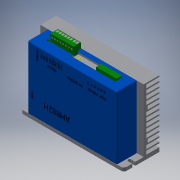
# Autodesk Inventor part: AM882
Saved by Autodesk Inventor 2016 (Build 200138000, 138)
## iProperties
Created: 2015-09-27
Part Number: AM882
Material: Generic
Document SubType Name: Modeling
Density: 1 g/cm^3
Appearance: Default
Autodesk Inventor part; units mm, degrees
ref_plane "YZ Plane" through (0, 0, 0) normal (1, 0, 0) x (0, 1, 0)
ref_plane "XZ Plane" through (0, 0, 0) normal (0, 1, 0) x (-1, 0, 0)
ref_plane "XY Plane" through (0, 0, 0) normal (0, 0, 1) x (1, 0, 0)
sketch "Sketch1" plane through (0, 0, 0) normal (0, 0, 1) x (1, 0, 0)
  line L0 (75.5, -37.5) -> (-75.5, -37.5)
  line L1 (-71.5, 14.5) -> (71.5, 14.5)
  arc A0 (-69.5, -2.25) -> (-69.5, 2.25) centre (-69.5, 0) ccw
  arc A1 (69.5, 2.25) -> (69.5, -2.25) centre (69.5, 0) ccw
  line L2 (-69.5, 2.25) -> (-75.5, 2.25)
  line L3 (-69.5, -2.25) -> (-75.5, -2.25)
  line L4 (69.5, 2.25) -> (75.5, 2.25)
  line L5 (69.5, -2.25) -> (75.5, -2.25)
  line L6 (75.5, 10.5) -> (75.5, 2.25)
  line L7 (75.5, -2.25) -> (75.5, -33.5)
  line L8 (-75.5, -37.5) -> (-75.5, -2.25)
  line L9 (-75.5, 2.25) -> (-75.5, 10.5)
  arc A2 (-71.5, 14.5) -> (-75.5, 10.5) centre (-71.5, 10.5) ccw
  arc A3 (75.5, 10.5) -> (71.5, 14.5) centre (71.5, 10.5) ccw
  line L10 (75.5, -2.25) -> (75.5, -37.5)
  point P0 (0, 0)
  dimension "d1" = 14.5
  dimension "d4" = 52
  dimension "d6" = 4.5
  dimension "d7" = 4.5
  dimension "d8" = 69.5
  dimension "d9" = 69.5
  dimension "d10" = 4
  dimension "d94" = 6
  dimension "d95" = 6
  constraints: 22 end point, 10 perpendicular, 8 point on circle, 8 tangent, 5 parallel, 4 centre point, 1 horizontal, 1 point on line
  measures "d1" distance from line of L1 point (0, 0)
  measures "d4" distance between parallel lines of L0 L1
  measures "d6" diameter of A0
  measures "d7" diameter of A1
  measures "d8" distance of point (0, 0) A1.centre
  measures "d9" distance of point (0, 0) A0.centre
  measures "d10" radius of A2
  measures "d94" distance from line of L9 A0.centre
  measures "d95" distance from line of L6 A1.centre
extrude "Extrusion1" add sketch "Sketch1" along normal blind 5
sketch "Sketch2" plane through (0, 0, 5) normal (0, 0, 1) x (1, 0, 0)
  line L0 (-75.5, -37.5) -> (-75.5, -2.25) projected
  arc A0 (69.5, 2.25) -> (69.5, -2.25) centre (69.5, 0) ccw projected
  line L1 (75.5, 10.5) -> (75.5, 2.25) projected
  line L2 (-71.5, 14.5) -> (71.5, 14.5) projected
  line L3 (-75.5, 2.25) -> (-75.5, 10.5) projected
  line L4 (-65.5, -14.5) -> (-65.5, 14.5)
  line L5 (65.5, -14.5) -> (65.5, 14.5)
  line L6 (-75.5, -14.5) -> (-65.5, -14.5)
  line L7 (65.5, -14.5) -> (75.5, -14.5)
  line L8 (75.5, -14.5) -> (75.5, -37.5)
  line L9 (-75.5, -14.5) -> (-75.5, -37.5)
  line L10 (-75.5, -37.5) -> (75.5, -37.5)
  point P0 (-71.5, -37.5)
  point P1 (0, 0)
  dimension "d13" = 14.5
  dimension "d15" = 10
  dimension "d16" = 10
  constraints: 14 end point, 3 perpendicular, 3 point on line, 1 parallel, 1 vertical
  measures "d13" distance from line of L2 A0.centre
  measures "d15" distance between parallel lines of L5 L1
  measures "d16" distance between parallel lines of L3 L4
extrude "Extrusion2" add sketch "Sketch2" along normal blind 92
sketch "Sketch3" plane through (0, 0, 97) normal (0, 0, 1) x (1, 0, 0)
  line L0 (65.5, 14.5) -> (65.5, -14.5) projected
  line L1 (-65.5, 14.5) -> (65.5, 14.5) projected
  line L2 (-65.5, -14.5) -> (-65.5, 14.5) projected
  line L3 (-65.5, -14.5) -> (65.5, -14.5)
  point P0 (0, 0)
  constraints: 2 end point, 1 perpendicular
extrude "Extrusion3" cut sketch "Sketch3" against normal blind 0.1
sketch "Sketch4" plane through (-71.5, 14.5, 0) normal (0, 1, 0) x (1, 0, 0)
  line L0 (6, -96.9) -> (137, -96.9) projected
  line L1 (137, -5) -> (137, -96.9) projected
  line L2 (0, -5) -> (143, -5) projected
  line L3 (6, -5) -> (6, -96.9) projected
  line L4 (6, -5) -> (137, -5)
  point P0 (71.5, 0)
  constraints: 2 end point, 1 collinear
extrude "Extrusion4" cut sketch "Sketch4" against normal blind 0.1
fillet "Fillet3" radius 2 5 edges at (-65.5, -0.05, 96.9) (0, 14.4, 96.9) (-65.5, 14.4, 50.95) (65.5, 14.4, 50.95) (65.5, -0.05, 96.9)
sketch "Sketch5" plane through (75.5, -37.5, 0) normal (1, 0, 0) x (0, 0, -1)
  line L0 (-5, 23.1496) -> (-97, 23.1496)
  line L1 (-0.1332, -0.4244) -> (-97.1332, -0.4244)
  line L2 (-95, -0.4244) -> (-90, -0.4244)
  line L3 (-90, -0.4244) -> (-90, 19.1496)
  line L4 (-90, 19.1496) -> (-95, 19.1496)
  line L5 (-95, 19.1496) -> (-95, -0.4244)
  line L6 (-97, 23.1496) -> (-97, 4.1496)
  line L7 (-88, -0.4244) -> (-83, -0.4244)
  line L8 (-83, -0.4244) -> (-83, 19.1496)
  line L9 (-83, 19.1496) -> (-88, 19.1496)
  line L10 (-88, 19.1496) -> (-88, -0.4244)
  line L11 (-76, -0.4244) -> (-81, -0.4244)
  line L12 (-81, -0.4244) -> (-81, 19.1496)
  line L13 (-81, 19.1496) -> (-76, 19.1496)
  line L14 (-76, 19.1496) -> (-76, -0.4244)
  line L15 (-69, -0.4244) -> (-74, -0.4244)
  line L16 (-74, -0.4244) -> (-74, 19.1496)
  line L17 (-74, 19.1496) -> (-69, 19.1496)
  line L18 (-69, 19.1496) -> (-69, -0.4244)
  line L19 (-67, -0.4244) -> (-62, -0.4244)
  line L20 (-62, -0.4244) -> (-62, 17.1496)
  line L21 (-62, 17.1496) -> (-67, 17.1496)
  line L22 (-67, 17.1496) -> (-67, -0.4244)
  line L23 (-55, -0.4244) -> (-60, -0.4244)
  line L24 (-60, -0.4244) -> (-60, 19.1496)
  line L25 (-60, 19.1496) -> (-55, 19.1496)
  line L26 (-55, 19.1496) -> (-55, -0.4244)
  line L27 (-48, -0.4244) -> (-53, -0.4244)
  line L28 (-53, -0.4244) -> (-53, 19.1496)
  line L29 (-53, 19.1496) -> (-48, 19.1496)
  line L30 (-48, 19.1496) -> (-48, -0.4244)
  line L31 (-46, -0.4244) -> (-41, -0.4244)
  line L32 (-41, -0.4244) -> (-41, 19.1496)
  line L33 (-41, 19.1496) -> (-46, 19.1496)
  line L34 (-46, 19.1496) -> (-46, -0.4244)
  line L35 (-34, -0.4244) -> (-39, -0.4244)
  line L36 (-39, -0.4244) -> (-39, 19.1496)
  line L37 (-39, 19.1496) -> (-34, 19.1496)
  line L38 (-34, 19.1496) -> (-34, -0.4244)
  line L39 (-27, -0.4244) -> (-32, -0.4244)
  line L40 (-32, -0.4244) -> (-32, 19.1496)
  line L41 (-32, 19.1496) -> (-27, 19.1496)
  line L42 (-27, 19.1496) -> (-27, -0.4244)
  line L43 (-20, -0.4244) -> (-25, -0.4244)
  line L44 (-25, -0.4244) -> (-25, 17.1496)
  line L45 (-25, 17.1496) -> (-20, 17.1496)
  line L46 (-20, 17.1496) -> (-20, -0.4244)
  line L47 (-13, -0.4244) -> (-18, -0.4244)
  line L48 (-18, -0.4244) -> (-18, 19.1496)
  line L49 (-18, 19.1496) -> (-13, 19.1496)
  line L50 (-13, 19.1496) -> (-13, -0.4244)
  line L51 (-6, -0.4244) -> (-11, -0.4244)
  line L52 (-11, -0.4244) -> (-11, 19.1496)
  line L53 (-11, 19.1496) -> (-6, 19.1496)
  line L54 (-6, 19.1496) -> (-6, -0.4244)
  point P0 (0, 33.5)
  dimension "d30" = 2
  dimension "d31" = 5
  dimension "d32" = 2
  dimension "d33" = 5
  dimension "d34" = 2
  dimension "d35" = 5
  dimension "d36" = 2
  dimension "d37" = 5
  dimension "d38" = 2
  dimension "d39" = 5
  dimension "d40" = 2
  dimension "d41" = 5
  dimension "d42" = 2
  dimension "d43" = 5
  dimension "d44" = 2
  dimension "d45" = 5
  dimension "d46" = 2
  dimension "d47" = 5
  dimension "d48" = 2
  dimension "d49" = 5
  dimension "d50" = 2
  dimension "d51" = 5
  dimension "d52" = 2
  dimension "d53" = 5
  dimension "d54" = 2
  dimension "d55" = 5
  dimension "d56" = 6
  dimension "d57" = 6
  constraints: 108 end point, 26 parallel, 13 horizontal, 13 perpendicular, 16 other
  measures "d30" distance between parallel lines of L6 L5
  measures "d31" distance between parallel lines of L3 L5
  measures "d32" distance between parallel lines of L3 L10
  measures "d33" distance between parallel lines of L8 L10
  measures "d34" distance between parallel lines of L8 L12
  measures "d35" distance between parallel lines of L14 L12
  measures "d36" distance between parallel lines of L14 L16
  measures "d37" distance between parallel lines of L18 L16
  measures "d38" distance between parallel lines of L18 L22
  measures "d39" distance between parallel lines of L20 L22
  measures "d40" distance between parallel lines of L20 L24
  measures "d41" distance between parallel lines of L26 L24
  measures "d42" distance between parallel lines of L26 L28
  measures "d43" distance between parallel lines of L30 L28
  measures "d44" distance between parallel lines of L30 L34
  measures "d45" distance between parallel lines of L34 L32
  measures "d46" distance between parallel lines of L32 L36
  measures "d47" distance between parallel lines of L38 L36
  measures "d48" distance between parallel lines of L38 L40
  measures "d49" distance between parallel lines of L42 L40
  measures "d50" distance between parallel lines of L42 L44
  measures "d51" distance between parallel lines of L46 L44
  measures "d52" distance between parallel lines of L46 L48
  measures "d53" distance between parallel lines of L50 L48
  measures "d54" distance between parallel lines of L52 L50
  measures "d55" distance between parallel lines of L54 L52
  measures "d56" distance between parallel lines of L0 L21
  measures "d57" distance between parallel lines of L0 L45
extrude "Extrusion5" cut sketch "Sketch5" against normal up to next
sketch "Sketch6" plane through (-75.5, -37.5, 67) normal (0, -1, 0) x (1, 0, 0)
  line L0 (46, 4.8951) -> (101, 4.8951)
  line L1 (101, 4.8951) -> (101, -51.0143)
  line L2 (101, -51.0143) -> (46, -51.0143)
  line L3 (46, -51.0143) -> (46, 4.8951)
  line L4 (0, -21) -> (0, -19) projected
  line L5 (151, -14) -> (151, -19) projected
  dimension "d66" = 46
  dimension "d67" = 50
  constraints: 8 end point, 2 parallel, 1 horizontal, 1 perpendicular
  measures "d66" distance between parallel lines of L4 L3
  measures "d67" distance between parallel lines of L5 L1
extrude "Extrusion7" cut sketch "Sketch6" against normal blind 16
sketch "Sketch7" plane through (-75.5, -21.5, 67) normal (0, -1, 0) x (1, 0, 0)
  line L0 (49, -48.5) -> (99, -48.5)
  line L1 (99, -48.5) -> (99, 1.5)
  line L2 (99, 1.5) -> (49, 1.5)
  line L3 (49, 1.5) -> (49, -48.5)
  line L4 (0, -67) -> (151, -67) projected
  line L5 (0, -12) -> (0, -7) projected
  point P0 (75.5, -67)
  dimension "d70" = 50
  dimension "d71" = 50
  dimension "d72" = 18.5
  dimension "d73" = 49
  constraints: 8 end point, 2 parallel, 1 horizontal, 1 perpendicular
  measures "d70" distance between parallel lines of L1 L3
  measures "d71" distance between parallel lines of L2 L0
  measures "d72" distance between parallel lines of L4 L0
  measures "d73" distance between parallel lines of L5 L3
extrude "Extrusion8" add sketch "Sketch7" along normal blind 14
sketch "Sketch8" plane through (65.5, -14.5, 5) normal (1, 0, 0) x (0, 0, -1)
  line L0 (-33, 18) -> (-20, 18)
  line L1 (-20, 18) -> (-20, 5)
  line L2 (-20, 5) -> (-33, 5)
  line L3 (-33, 5) -> (-33, 18)
  line L4 (0, 16.75) -> (0, 12.25) projected
  line L5 (0, 0) -> (-92, 0) projected
  point P0 (5, 14.5)
  dimension "d76" = 13
  dimension "d77" = 13
  dimension "d78" = 20
  dimension "d79" = 5
  constraints: 8 end point, 2 parallel, 1 horizontal, 1 perpendicular
  measures "d76" distance between parallel lines of L2 L0
  measures "d77" distance between parallel lines of L3 L1
  measures "d78" distance between parallel lines of L4 L1
  measures "d79" distance between parallel lines of L5 L2
extrude "Extrusion9" cut sketch "Sketch8" against normal blind 0.25
sketch "Sketch9" plane through (0, 0, 96.9) normal (0, 0, 1) x (1, 0, 0)
  circle A0 centre (50.5, -6.5) radius 1.5
  circle A1 centre (50.5, -0.5) radius 1.5
  line L0 (-75.5, -14.5) -> (75.5, -14.5) projected
  line L1 (47, -7.5) -> (13, -7.5)
  line L2 (13, -7.5) -> (13, -0.5)
  line L3 (13, -0.5) -> (47, -0.5)
  line L4 (47, -0.5) -> (47, -7.5)
  line L5 (65.5, -14.5) -> (65.5, 12.4) projected
  line L6 (13, -7.5) -> (-51, -7.5)
  line L7 (-51, -7.5) -> (-51, 2.5)
  line L8 (-51, 2.5) -> (13, 2.5)
  line L9 (13, 2.5) -> (13, -7.5)
  point P0 (0, 0)
  dimension "d82" = 3
  dimension "d83" = 3
  dimension "d84" = 8
  dimension "d85" = 14
  dimension "d86" = 7
  dimension "d87" = 7
  dimension "d88" = 18.5
  dimension "d89" = 15
  dimension "d90" = 15
  dimension "d91" = 34
  dimension "d92" = 10
  dimension "d93" = 64
  constraints: 16 end point, 4 parallel, 2 centre point, 2 horizontal, 2 perpendicular
  measures "d82" diameter of A0
  measures "d83" diameter of A1
  measures "d84" distance from line of L0 A0.centre
  measures "d85" distance from line of L0 A1.centre
  measures "d86" distance between parallel lines of L1 L3
  measures "d87" distance between parallel lines of L0 L1
  measures "d88" distance between parallel lines of L5 L4
  measures "d89" distance from line of L5 A0.centre
  measures "d90" distance from line of L5 A1.centre
  measures "d91" distance between parallel lines of L2 L4
  measures "d92" distance between parallel lines of L8 L6
  measures "d93" distance between parallel lines of L7 L2
extrude "Extrusion10" cut sketch "Sketch9" against normal blind 2.5
sketch "Sketch10" plane through (0, 0, 94.4) normal (0, 0, 1) x (1, 0, 0)
  line L0 (47, -7.5) -> (-51, -7.5) projected
  line L1 (13, 2.5) -> (13, -0.5) projected
  line L2 (-51, -7.5) -> (-21, -7.5)
  line L3 (-21, -7.5) -> (-21, 0.5)
  line L4 (-21, 0.5) -> (-51, 0.5)
  line L5 (-51, 0.5) -> (-51, -7.5)
  line L6 (13, -0.5) -> (47, -0.5) projected
  line L7 (47, -7.5) -> (13.25, -7.5)
  line L8 (13.25, -7.5) -> (13.25, -0.5)
  line L9 (13.25, -0.5) -> (47, -0.5)
  line L10 (47, -0.5) -> (47, -7.5)
  point P0 (0, 0)
  dimension "d98" = 8
  dimension "d99" = 30
  dimension "d118" = 0.25
  constraints: 16 end point, 4 parallel, 2 horizontal, 2 perpendicular, 1 point on line
  measures "d98" distance between parallel lines of L0 L4
  measures "d99" distance between parallel lines of L5 L3
  measures "d118" distance between parallel lines of L1 L8
extrude "Extrusion11" add sketch "Sketch10" along normal blind 5
sketch "Sketch11" plane through (-75.5, -35.5, 67) normal (0, -1, 0) x (1, 0, 0)
  circle A0 centre (74, -23.5) radius 20.5
  line L0 (49, 1.5) -> (49, -48.5) projected
  line L1 (49, -48.5) -> (99, -48.5) projected
  circle A1 centre (74, -23.5) radius 18.5
  circle A2 centre (74, -23.5) radius 14.5
  circle A3 centre (74, -23.5) radius 12.5
  circle A4 centre (74, -23.5) radius 8.5
  circle A5 centre (74, -23.5) radius 6.5
  point P0 (75.5, -67)
  dimension "d102" = 25
  dimension "d103" = 25
  dimension "d104" = 41
  dimension "d105" = 2
  dimension "d106" = 4
  dimension "d107" = 2
  dimension "d108" = 4
  dimension "d109" = 2
  constraints: 6 centre point
  measures "d102" distance from line of A0.centre L0
  measures "d103" distance from line of L1 A0.centre
  measures "d104" diameter of A0
  measures "d105" radial gap between concentric circles of A0 A1
  measures "d106" radial gap between concentric circles of A1 A2
  measures "d107" radial gap between concentric circles of A2 A3
  measures "d108" radial gap between concentric circles of A3 A4
  measures "d109" radial gap between concentric circles of A4 A5
extrude "Extrusion12" add sketch "Sketch11" along normal blind 2
fillet "Fillet4" radius 1 6 edges at (-22, -37.5, 43.5) (-20, -37.5, 43.5) (-16, -37.5, 43.5) (-14, -37.5, 43.5) (-10, -37.5, 43.5) (-8, -37.5, 43.5)
sketch "Sketch12" plane through (0, 0, 99.4) normal (0, 0, 1) x (1, 0, 0)
  line L0 (47, -0.5) -> (13.25, -0.5) projected
  line L1 (47, -0.5) -> (13.25, -0.5)
  line L2 (13.25, -0.5) -> (13.25, -11.5)
  line L3 (13.25, -11.5) -> (47, -11.5)
  line L4 (47, -11.5) -> (47, -0.5)
  point P0 (-51, -7.5)
  point P1 (13, -0.5)
  dimension "d120" = 11
  constraints: 8 end point, 2 parallel, 1 horizontal, 1 perpendicular
  measures "d120" distance between parallel lines of L3 L0
extrude "Extrusion13" add sketch "Sketch12" along normal blind 8
sketch "Sketch13" plane through (0, 0, 107.4) normal (0, 0, 1) x (1, 0, 0)
  line L0 (14.25, -10.5) -> (17.25, -10.5)
  line L1 (17.25, -10.5) -> (17.25, -6.5)
  line L2 (17.25, -6.5) -> (14.25, -6.5)
  line L3 (14.25, -6.5) -> (14.25, -10.5)
  line L4 (13.25, -11.5) -> (47, -11.5) projected
  line L5 (13.25, -0.5) -> (13.25, -11.5) projected
  line L6 (18.25, -6.5) -> (21.25, -6.5)
  line L7 (21.25, -6.5) -> (21.25, -10.5)
  line L8 (21.25, -10.5) -> (18.25, -10.5)
  line L9 (18.25, -10.5) -> (18.25, -6.5)
  line L10 (23, -6.5) -> (26, -6.5)
  line L11 (26, -6.5) -> (26, -10.5)
  line L12 (26, -10.5) -> (23, -10.5)
  line L13 (23, -10.5) -> (23, -6.5)
  line L14 (27, -6.5) -> (30, -6.5)
  line L15 (30, -6.5) -> (30, -10.5)
  line L16 (30, -10.5) -> (27, -10.5)
  line L17 (27, -10.5) -> (27, -6.5)
  line L18 (31, -6.5) -> (34, -6.5)
  line L19 (34, -6.5) -> (34, -10.5)
  line L20 (34, -10.5) -> (31, -10.5)
  line L21 (31, -10.5) -> (31, -6.5)
  line L22 (35, -6.5) -> (38, -6.5)
  line L23 (38, -6.5) -> (38, -10.5)
  line L24 (38, -10.5) -> (35, -10.5)
  line L25 (35, -10.5) -> (35, -6.5)
  line L26 (39, -6.5) -> (42, -6.5)
  line L27 (42, -6.5) -> (42, -10.5)
  line L28 (42, -10.5) -> (39, -10.5)
  line L29 (39, -10.5) -> (39, -6.5)
  line L30 (43, -6.5) -> (46, -6.5)
  line L31 (46, -6.5) -> (46, -10.5)
  line L32 (46, -10.5) -> (43, -10.5)
  line L33 (43, -10.5) -> (43, -6.5)
  line L34 (47, -11.5) -> (47, -0.5) projected
  point P0 (0, 0)
  dimension "d121" = 1
  dimension "d122" = 1
  dimension "d123" = 3
  dimension "d124" = 4
  dimension "d125" = 3
  dimension "d126" = 3
  dimension "d127" = 3
  dimension "d128" = 3
  dimension "d129" = 3
  dimension "d130" = 3
  dimension "d131" = 3
  dimension "d132" = 1
  dimension "d133" = 1
  dimension "d134" = 1.75
  dimension "d135" = 1
  dimension "d136" = 1
  dimension "d137" = 1
  dimension "d138" = 1
  dimension "d139" = 1
  constraints: 64 end point, 16 parallel, 12 point on line, 8 horizontal, 8 perpendicular
  measures "d121" distance between parallel lines of L4 L0
  measures "d122" distance between parallel lines of L5 L3
  measures "d123" distance between parallel lines of L1 L3
  measures "d124" distance between parallel lines of L2 L0
  measures "d125" distance of L7.end L8.end
  measures "d126" distance of L11.end L12.end
  measures "d127" distance of L15.end L16.end
  measures "d128" distance of L19.end L20.end
  measures "d129" distance of L23.end L24.end
  measures "d130" distance of L27.end L28.end
  measures "d131" distance between parallel lines of L31 L33
  measures "d132" distance between parallel lines of L27 L33
  measures "d133" distance between parallel lines of L1 L9
  measures "d134" distance between parallel lines of L13 L7
  measures "d135" distance between parallel lines of L17 L11
  measures "d136" distance between parallel lines of L21 L15
  measures "d137" distance between parallel lines of L19 L25
  measures "d138" distance between parallel lines of L29 L23
  measures "d139" distance between parallel lines of L34 L31
extrude "Extrusion14" cut sketch "Sketch13" against normal blind 0.25
sketch "Sketch14" plane through (13.25, -0.5, 96.9) normal (0, 1, 0) x (1, 0, 0)
  circle A0 centre (31.25, -6.5) radius 1.25
  circle A1 centre (27.25, -6.5) radius 1.25
  circle A2 centre (23.25, -6.5) radius 1.25
  line L0 (32.75, -10.5) -> (32.75, -10.25) projected
  line L1 (28.75, -10.5) -> (28.75, -10.25) projected
  line L2 (24.75, -10.5) -> (24.75, -10.25) projected
  circle A3 centre (19.25, -6.5) radius 1.25
  circle A4 centre (15.25, -6.5) radius 1.25
  circle A5 centre (11.25, -6.5) radius 1.25
  circle A6 centre (6.5, -6.5) radius 1.25
  circle A7 centre (2.5, -6.5) radius 1.25
  line L3 (20.75, -10.5) -> (20.75, -10.25) projected
  line L4 (16.75, -10.5) -> (16.75, -10.25) projected
  line L5 (12.75, -10.5) -> (12.75, -10.25) projected
  line L6 (8, -10.5) -> (8, -10.25) projected
  line L7 (4, -10.5) -> (4, -10.25) projected
  line L8 (33.75, -10.5) -> (0, -10.5) projected
  point P0 (-13.25, 96.9)
  dimension "d142" = 2.5
  dimension "d143" = 2.5
  dimension "d144" = 2.5
  dimension "d145" = 1.5
  dimension "d146" = 1.5
  dimension "d147" = 1.5
  dimension "d148" = 2.5
  dimension "d149" = 2.5
  dimension "d150" = 2.5
  dimension "d151" = 2.5
  dimension "d152" = 2.5
  dimension "d153" = 1.5
  dimension "d154" = 1.5
  dimension "d155" = 1.5
  dimension "d156" = 1.5
  dimension "d157" = 1.5
  dimension "d160" = 4
  dimension "d161" = 4
  dimension "d162" = 4
  dimension "d163" = 4
  dimension "d164" = 4
  dimension "d165" = 4
  dimension "d166" = 4
  dimension "d167" = 4
  constraints: 8 centre point, 1 other
  measures "d142" diameter of A0
  measures "d143" diameter of A1
  measures "d144" diameter of A2
  measures "d145" distance from line of L0 A0.centre
  measures "d146" distance from line of L1 A1.centre
  measures "d147" distance from line of A2.centre L2
  measures "d148" diameter of A3
  measures "d149" diameter of A4
  measures "d150" diameter of A5
  measures "d151" diameter of A6
  measures "d152" diameter of A7
  measures "d153" distance from line of L3 A3.centre
  measures "d154" distance from line of L4 A4.centre
  measures "d155" distance from line of L5 A5.centre
  measures "d156" distance from line of L6 A6.centre
  measures "d157" distance from line of L7 A7.centre
extrude "Extrusion15" cut sketch "Sketch14" against normal blind 0.25
sketch "Sketch15" plane through (0, 0, 94.4) normal (0, 0, 1) x (1, 0, 0)
  circle A0 centre (7, -2.5) radius 2
  line L0 (13.25, -7.5) -> (-21, -7.5) projected
  line L1 (13, 2.5) -> (13, -0.5) projected
  point P0 (0, 0)
  dimension "d168" = 4
  dimension "d169" = 5
  dimension "d170" = 6
  constraints: 1 centre point
  measures "d168" diameter of A0
  measures "d169" distance from line of L0 A0.centre
  measures "d170" distance from line of A0.centre L1
extrude "Extrusion16" add sketch "Sketch15" along normal blind 0.25
sketch "Sketch16" plane through (-71.5, 14.4, 0) normal (0, 1, 0) x (1, 0, 0)
  line L0 (124.0205, -77.7142) -> (124.0205, -93.0848) construction
  line L1 (124.0205, -93.0848) -> (120.6087, -93.0848) construction
  line L2 (120.6087, -93.0848) -> (120.6087, -77.7142) construction
  line L3 (120.6087, -77.7142) -> (124.0205, -77.7142) construction
  line L4 (117.7292, -83.7972) -> (117.7292, -99.1678) construction
  line L5 (117.7292, -99.1678) -> (114.3173, -99.1678) construction
  line L6 (114.3173, -99.1678) -> (114.3173, -83.7972) construction
  line L7 (114.3173, -83.7972) -> (117.7292, -83.7972) construction
  line L8 (113.677, -83.7972) -> (113.677, -99.1678) construction
  line L9 (113.677, -99.1678) -> (110.2651, -99.1678) construction
  line L10 (110.2651, -99.1678) -> (110.2651, -83.7972) construction
  line L11 (110.2651, -83.7972) -> (113.677, -83.7972) construction
  line L12 (109.6248, -83.7972) -> (109.6248, -99.1678) construction
  line L13 (109.6248, -99.1678) -> (106.2129, -99.1678) construction
  line L14 (106.2129, -99.1678) -> (106.2129, -83.7972) construction
  line L15 (106.2129, -83.7972) -> (109.6248, -83.7972) construction
  line L16 (105.5015, -83.7972) -> (105.5015, -99.1678) construction
  line L17 (105.5015, -99.1678) -> (102.0896, -99.1678) construction
  line L18 (102.0896, -99.1678) -> (102.0896, -83.7972) construction
  line L19 (102.0896, -83.7972) -> (105.5015, -83.7972) construction
  line L20 (101.5204, -83.7972) -> (101.5204, -99.1678) construction
  line L21 (101.5204, -99.1678) -> (98.1085, -99.1678) construction
  line L22 (98.1085, -99.1678) -> (98.1085, -83.7972) construction
  line L23 (98.1085, -83.7972) -> (101.5204, -83.7972) construction
  line L24 (97.5392, -83.7972) -> (97.5392, -99.1678) construction
  line L25 (97.5392, -99.1678) -> (94.1274, -99.1678) construction
  line L26 (94.1274, -99.1678) -> (94.1274, -83.7972) construction
  line L27 (94.1274, -83.7972) -> (97.5392, -83.7972) construction
  line L28 (92.6339, -83.7972) -> (92.6339, -99.1678) construction
  line L29 (92.6339, -99.1678) -> (89.2221, -99.1678) construction
  line L30 (89.2221, -99.1678) -> (89.2221, -83.7972) construction
  line L31 (89.2221, -83.7972) -> (92.6339, -83.7972) construction
  line L32 (88.5817, -83.7972) -> (88.5817, -99.1678) construction
  line L33 (88.5817, -99.1678) -> (85.1699, -99.1678) construction
  line L34 (85.1699, -99.1678) -> (85.1699, -83.7972) construction
  line L35 (85.1699, -83.7972) -> (88.5817, -83.7972) construction
  line L36 (46.4174, -85.3632) -> (49.8292, -85.3632) construction
  line L37 (49.8292, -85.3632) -> (49.8292, -100.7338) construction
  line L38 (49.8292, -100.7338) -> (46.4174, -100.7338) construction
  line L39 (46.4174, -100.7338) -> (46.4174, -85.3632) construction
  line L40 (40.9745, -85.4501) -> (44.3863, -85.4501) construction
  line L41 (44.3863, -85.4501) -> (44.3863, -100.8207) construction
  line L42 (44.3863, -100.8207) -> (40.9745, -100.8207) construction
  line L43 (40.9745, -100.8207) -> (40.9745, -85.4501) construction
  line L44 (36.3138, -85.3632) -> (39.7257, -85.3632) construction
  line L45 (39.7257, -85.3632) -> (39.7257, -100.7338) construction
  line L46 (39.7257, -100.7338) -> (36.3138, -100.7338) construction
  line L47 (36.3138, -100.7338) -> (36.3138, -85.3632) construction
  line L48 (31.7559, -85.3838) -> (35.1678, -85.3838) construction
  line L49 (35.1678, -85.3838) -> (35.1678, -100.7544) construction
  line L50 (35.1678, -100.7544) -> (31.7559, -100.7544) construction
  line L51 (31.7559, -100.7544) -> (31.7559, -85.3838) construction
  line L52 (26.9925, -85.3154) -> (30.4044, -85.3154) construction
  line L53 (30.4044, -85.3154) -> (30.4044, -100.686) construction
  line L54 (30.4044, -100.686) -> (26.9925, -100.686) construction
  line L55 (26.9925, -100.686) -> (26.9925, -85.3154) construction
  line L56 (22.403, -85.4023) -> (25.8148, -85.4023) construction
  line L57 (25.8148, -85.4023) -> (25.8148, -100.7729) construction
  line L58 (25.8148, -100.7729) -> (22.403, -100.7729) construction
  line L59 (22.403, -100.7729) -> (22.403, -85.4023) construction
  line L60 (131.3809, -26.5906) -> (131.3809, -41.9612) construction
  line L61 (131.3809, -41.9612) -> (127.969, -41.9612) construction
  line L62 (127.969, -41.9612) -> (127.969, -26.5906) construction
  line L63 (127.969, -26.5906) -> (131.3809, -26.5906) construction
  line L64 (94.9849, -76.7544) -> (110.3555, -76.7544) construction
  line L65 (110.3555, -76.7544) -> (110.3555, -81.8669) construction
  line L66 (110.3555, -81.8669) -> (94.9849, -81.8669) construction
  line L67 (94.9849, -81.8669) -> (94.9849, -76.7544) construction
  line L68 (56.4352, -81.8669) -> (56.4352, -76.7544) construction
  line L69 (56.4352, -76.7544) -> (78.8967, -76.7544) construction
  line L70 (78.8967, -76.7544) -> (78.8967, -81.8669) construction
  line L71 (78.8967, -81.8669) -> (56.4352, -81.8669) construction
  line L72 (22.1005, -82.0358) -> (22.1005, -76.9232) construction
  line L73 (22.1005, -76.9232) -> (49.7959, -76.9232) construction
  line L74 (49.7959, -76.9232) -> (49.7959, -82.0358) construction
  line L75 (49.7959, -82.0358) -> (22.1005, -82.0358) construction
  line L76 (75.3116, -27.3787) -> (75.3116, -22.2661) construction
  line L77 (75.3116, -22.2661) -> (90.6822, -22.2661) construction
  line L78 (90.6822, -22.2661) -> (90.6822, -27.3787) construction
  line L79 (90.6822, -27.3787) -> (75.3116, -27.3787) construction
  constraints: 40 other
body "Solid1"
